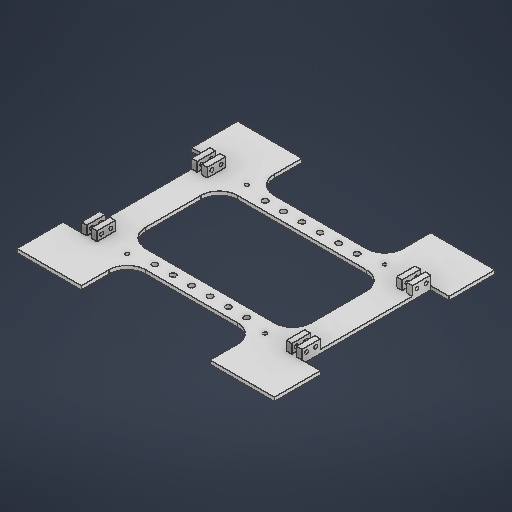
# Autodesk Inventor part: base
Saved by Autodesk Inventor 2026.1 (Build 301233000, 233)
## iProperties
Created: 2025-10-16
Part Number: base
Material: Generic
Document SubType Name: Modeling
Designer: emanuel
Density: 1 g/cm^3
Appearance: Default
Author: emanuel
Autodesk Inventor part; units mm, degrees
ref_plane "YZ Plane" through (0, 0, 0) normal (1, 0, 0) x (0, 1, 0)
ref_plane "XZ Plane" through (0, 0, 0) normal (0, 1, 0) x (-1, 0, 0)
ref_plane "XY Plane" through (0, 0, 0) normal (0, 0, 1) x (1, 0, 0)
sketch "Sketch1" plane through (0, 0, 0) normal (0, 1, 0) x (-1, 0, 0)
  line L0 (0, 0) -> (140, 0)
  line L1 (140, 0) -> (140, -120)
  line L2 (140, -120) -> (0, -120)
  line L3 (0, -120) -> (0, 0)
  line L4 (140, 0) -> (0, 0)
  line L5 (0, 0) -> (0, -25)
  line L6 (0, -25) -> (140, -25)
  line L7 (140, -25) -> (140, 0)
  line L8 (140, -120) -> (0, -120)
  line L9 (0, -120) -> (0, -95)
  line L10 (0, -95) -> (140, -95)
  line L11 (140, -95) -> (140, -120)
  line L12 (140, -25) -> (130, -25)
  line L13 (130, -25) -> (130, -95)
  line L14 (130, -95) -> (140, -95)
  line L15 (140, -95) -> (140, -25)
  line L16 (0, -25) -> (10, -25)
  line L17 (10, -25) -> (10, -95)
  line L18 (10, -95) -> (0, -95)
  line L19 (0, -95) -> (0, -25)
  line L20 (130, -25) -> (115, -25)
  line L21 (115, -25) -> (115, -95)
  line L22 (115, -95) -> (130, -95)
  line L23 (130, -95) -> (130, -25)
  line L24 (10, -95) -> (25, -95)
  line L25 (25, -95) -> (25, -25)
  line L26 (25, -25) -> (10, -25)
  line L27 (10, -25) -> (10, -95)
  line L28 (115, -25) -> (25, -25)
  line L29 (25, -25) -> (25, -35)
  line L30 (25, -35) -> (115, -35)
  line L31 (115, -35) -> (115, -25)
  line L32 (115, -95) -> (25, -95)
  line L33 (25, -95) -> (25, -85)
  line L34 (25, -85) -> (115, -85)
  line L35 (115, -85) -> (115, -95)
  line L36 (115, -30) -> (25, -30)
  line L37 (115, -90) -> (25, -90)
  line L38 (115, -30) -> (105, -30)
  line L39 (105, -30) -> (95, -30)
  line L40 (95, -30) -> (85, -30)
  line L41 (85, -30) -> (75, -30)
  line L42 (75, -30) -> (65, -30)
  line L43 (65, -30) -> (55, -30)
  line L44 (55, -30) -> (45, -30)
  line L45 (45, -30) -> (35, -30)
  line L46 (115, -90) -> (105, -90)
  line L47 (105, -90) -> (95, -90)
  line L48 (95, -90) -> (85, -90)
  line L49 (85, -90) -> (75, -90)
  line L50 (75, -90) -> (65, -90)
  line L51 (65, -90) -> (55, -90)
  line L52 (55, -90) -> (45, -90)
  line L53 (45, -90) -> (35, -90)
  line L54 (35, -90) -> (25, -90)
  circle A0 centre (105, -30) radius 1.5
  circle A1 centre (95, -30) radius 1.5
  circle A2 centre (85, -30) radius 1.5
  circle A3 centre (75, -30) radius 1.5
  circle A4 centre (65, -30) radius 1.5
  circle A5 centre (55, -30) radius 1.5
  circle A6 centre (45, -30) radius 1.5
  circle A7 centre (35, -30) radius 1.5
  circle A8 centre (105, -90) radius 1.5
  circle A9 centre (95, -90) radius 1.5
  circle A10 centre (85, -90) radius 1.5
  circle A11 centre (75, -90) radius 1.5
  circle A12 centre (65, -90) radius 1.5
  circle A13 centre (55, -90) radius 1.5
  circle A14 centre (45, -90) radius 1.5
  circle A15 centre (35, -90) radius 1.5
  line L55 (140, 0) -> (105, 0)
  line L56 (105, 0) -> (105, -25)
  line L57 (105, -25) -> (140, -25)
  line L58 (140, -25) -> (140, 0)
  line L59 (140, -95) -> (105, -95)
  line L60 (105, -95) -> (105, -120)
  line L61 (105, -120) -> (140, -120)
  line L62 (140, -120) -> (140, -95)
  line L63 (0, 0) -> (35, 0)
  line L64 (35, 0) -> (35, -25)
  line L65 (35, -25) -> (0, -25)
  line L66 (0, -25) -> (0, 0)
  line L67 (0, -95) -> (35, -95)
  line L68 (35, -95) -> (35, -120)
  line L69 (35, -120) -> (0, -120)
  line L70 (0, -120) -> (0, -95)
  dimension "d0" = 140
  dimension "d1" = 120
  dimension "d2" = 25
  dimension "d3" = 25
  dimension "d4" = 10
  dimension "d5" = 10
  dimension "d6" = 15
  dimension "d7" = 15
  dimension "d8" = 10
  dimension "d9" = 10
  dimension "d10" = 10
  dimension "d11" = 10
  dimension "d12" = 10
  dimension "d13" = 10
  dimension "d14" = 10
  dimension "d15" = 10
  dimension "d16" = 10
  dimension "d17" = 10
  dimension "d18" = 10
  dimension "d19" = 10
  dimension "d20" = 10
  dimension "d21" = 10
  dimension "d22" = 10
  dimension "d23" = 10
  dimension "d24" = 10
  dimension "d25" = 10
  dimension "d26" = 10
  dimension "d27" = 3
  dimension "d28" = 3
  dimension "d29" = 3
  dimension "d30" = 3
  dimension "d31" = 3
  dimension "d32" = 3
  dimension "d33" = 3
  dimension "d34" = 3
  dimension "d35" = 3
  dimension "d36" = 3
  dimension "d37" = 3
  dimension "d38" = 3
  dimension "d39" = 3
  dimension "d40" = 3
  dimension "d41" = 3
  dimension "d42" = 3
  dimension "d43" = 35
  dimension "d44" = 35
  dimension "d45" = 35
  dimension "d46" = 35
  constraints: 138 end point, 27 equal length, 16 centre point, 16 coincident, 13 horizontal, 13 perpendicular, 12 point on line, 4 midpoint, 22 other
  measures "d0" distance of L1.end L2.end
  measures "d1" distance of L0.end L1.end
  measures "d2" distance of L5.end L4.end
  measures "d3" distance of L8.end L9.end
  measures "d4" distance of L14.end L13.end
  measures "d5" distance of L17.end L18.end
  measures "d6" distance of L22.end L21.end
  measures "d7" distance of L26.end L25.end
  measures "d8" distance of L29.end L28.end
  measures "d9" distance of L32.end L33.end
  measures "d10" distance of L38.start L38.end
  measures "d11" distance of L38.end L39.end
  measures "d12" distance of L39.end L40.end
  measures "d13" distance of L40.end L41.end
  measures "d14" distance of L41.end L42.end
  measures "d15" distance of L42.end L43.end
  measures "d16" distance of L43.end L44.end
  measures "d17" distance of L44.end L45.end
  measures "d18" distance of L46.start L46.end
  measures "d19" distance of L46.end L47.end
  measures "d20" distance of L47.end L48.end
  measures "d21" distance of L48.end L49.end
  measures "d22" distance of L49.end L50.end
  measures "d23" distance of L50.end L51.end
  measures "d24" distance of L51.end L52.end
  measures "d25" distance of L52.end L53.end
  measures "d26" distance of L53.end L54.end
  measures "d27" diameter of A0
  measures "d28" diameter of A1
  measures "d29" diameter of A2
  measures "d30" diameter of A3
  measures "d31" diameter of A4
  measures "d32" diameter of A5
  measures "d33" diameter of A6
  measures "d34" diameter of A7
  measures "d35" diameter of A8
  measures "d36" diameter of A9
  measures "d37" diameter of A10
  measures "d38" diameter of A11
  measures "d39" diameter of A12
  measures "d40" diameter of A13
  measures "d41" diameter of A14
  measures "d42" diameter of A15
  measures "d43" distance of L57.end L56.end
  measures "d44" distance of L61.end L60.end
  measures "d45" distance of L64.end L65.end
  measures "d46" distance of L68.end L69.end
extrude "Extrusion1" add sketch "Sketch1" along normal blind 2 contours L0 L64 L6 L3 | L0 L1 L6 L56 | L6 L21 L36 A0 A1 A2 A3 A4 A5 A6 A7 L25 | L10 L68 L2 L3 | L6 L25 L10 L17 | L6 L13 L10 L21 | L36 A7 A6 A5 A4 A3 A2 A1 A0 L21 L30 L25 | L25 L37 A15 A14 A13 A12 A11 A10 A9 A8 L21 L10 | L1 L2 L60 L10 | A7 L36 | L36 A7 | L25 L34 L21 L37 A8 A9 A10 A11 A12 A13 A14 A15 | A0 L36 | L36 A0 | A15 L37 | L37 A15 | A8 L37 | L37 A8
fillet "Fillet1" radius 10 8 edges at (-105, 1, -25) (-115, 1, -85) (-25, 1, -85) (-25, 1, -35) (-115, 1, -35) (-35, 1, -95) (-105, 1, -95) (-35, 1, -25)
sketch "Sketch2" plane through (0, 2, 0) normal (0, 1, 0) x (1, 0, 0)
  line L0 (-130, 95) -> (-130, 25) projected
  line L1 (-130, 25) -> (-127, 25)
  line L2 (-127, 25) -> (-127, 95)
  line L3 (-127, 95) -> (-130, 95)
  line L4 (-130, 95) -> (-130, 25)
  line L5 (-127, 25) -> (-124.5, 25)
  line L6 (-124.5, 25) -> (-124.5, 95)
  line L7 (-124.5, 95) -> (-127, 95)
  line L8 (-127, 95) -> (-127, 25)
  line L9 (-124.5, 25) -> (-121.5, 25)
  line L10 (-121.5, 25) -> (-121.5, 95)
  line L11 (-121.5, 95) -> (-124.5, 95)
  line L12 (-124.5, 95) -> (-124.5, 25)
  line L13 (-10, 25) -> (-10, 95) projected
  line L14 (-10, 25) -> (-13, 25)
  line L15 (-13, 25) -> (-13, 95)
  line L16 (-13, 95) -> (-10, 95)
  line L17 (-10, 95) -> (-10, 25)
  line L18 (-13, 25) -> (-15.5, 25)
  line L19 (-15.5, 25) -> (-15.5, 95)
  line L20 (-15.5, 95) -> (-13, 95)
  line L21 (-13, 95) -> (-13, 25)
  line L22 (-15.5, 25) -> (-18.5, 25)
  line L23 (-18.5, 25) -> (-18.5, 95)
  line L24 (-18.5, 95) -> (-15.5, 95)
  line L25 (-15.5, 95) -> (-15.5, 25)
  line L26 (-130, 25) -> (-121.5, 25)
  line L27 (-121.5, 25) -> (-121.5, 35)
  line L28 (-121.5, 35) -> (-130, 35)
  line L29 (-130, 35) -> (-130, 25)
  line L30 (-130, 95) -> (-121.5, 95)
  line L31 (-121.5, 95) -> (-121.5, 85)
  line L32 (-121.5, 85) -> (-130, 85)
  line L33 (-130, 85) -> (-130, 95)
  line L34 (-18.5, 25) -> (-10, 25)
  line L35 (-10, 25) -> (-10, 35)
  line L36 (-10, 35) -> (-18.5, 35)
  line L37 (-18.5, 35) -> (-18.5, 25)
  line L38 (-18.5, 95) -> (-10, 95)
  line L39 (-10, 95) -> (-10, 85)
  line L40 (-10, 85) -> (-18.5, 85)
  line L41 (-18.5, 85) -> (-18.5, 95)
  line L42 (-130, 25) -> (-127, 25)
  line L43 (-127, 25) -> (-127, 35)
  line L44 (-127, 35) -> (-130, 35)
  line L45 (-130, 35) -> (-130, 25)
  line L46 (-18.5, 25) -> (-15.5, 25)
  line L47 (-15.5, 25) -> (-15.5, 35)
  line L48 (-15.5, 35) -> (-18.5, 35)
  line L49 (-18.5, 35) -> (-18.5, 25)
  point P0 (0, 0)
  point P1 (-124.5, 35)
  point P2 (-124.5, 85)
  point P3 (-127, 85)
  point P4 (-13, 35)
  point P5 (-13, 85)
  point P6 (-15.5, 85)
  dimension "d50" = 3
  dimension "d51" = 2.5
  dimension "d52" = 3
  dimension "d53" = 3
  dimension "d54" = 2.5
  dimension "d55" = 3
  dimension "d56" = 10
  dimension "d57" = 10
  dimension "d58" = 10
  dimension "d59" = 10
  constraints: 96 end point, 24 parallel, 13 point on line, 12 horizontal, 12 perpendicular
  measures "d50" distance of L3.end L2.end
  measures "d51" distance of L7.end L6.end
  measures "d52" distance of L11.end L10.end
  measures "d53" distance of L15.end L16.end
  measures "d54" distance of L19.end L20.end
  measures "d55" distance of L23.end L24.end
  measures "d56" distance of L27.end L26.end
  measures "d57" distance of L30.end L31.end
  measures "d58" distance of L35.end L34.end
  measures "d59" distance of L38.end L39.end
extrude "Extrusion2" add sketch "Sketch2" along normal blind 5 contours L3 L2 L32 L0 | L28 L2 L1 L0 | L11 L10 L32 L6 | L28 L10 L9 L6 | L14 L15 L36 L13 | L40 L15 L16 L13 | L22 L23 L36 L19 | L40 L23 L24 L19
sketch "Sketch3" plane through (-10, 0, -25) normal (1, 0, 0) x (0, 0, -1)
  line L0 (0, 7) -> (10, 7) projected
  line L1 (0, 7) -> (2.5, 7)
  line L2 (2.5, 7) -> (2.5, 4.5)
  line L3 (2.5, 4.5) -> (0, 4.5)
  line L4 (0, 4.5) -> (0, 7)
  line L5 (2.5, 4.5) -> (7.5, 4.5)
  circle A0 centre (2.5, 4.5) radius 1
  circle A1 centre (7.5, 4.5) radius 1
  line L6 (60, 7) -> (70, 7) projected
  line L7 (60, 7) -> (62.5, 7)
  line L8 (62.5, 7) -> (62.5, 4.5)
  line L9 (62.5, 4.5) -> (60, 4.5)
  line L10 (60, 4.5) -> (60, 7)
  line L11 (62.5, 4.5) -> (67.5, 4.5)
  circle A2 centre (67.5, 4.5) radius 1
  circle A3 centre (62.5, 4.5) radius 1
  point P0 (-25, 0)
  dimension "d62" = 2.5
  dimension "d63" = 2.5
  dimension "d64" = 5
  dimension "d65" = 2
  dimension "d66" = 2
  dimension "d67" = 2.5
  dimension "d68" = 2.5
  dimension "d69" = 5
  dimension "d70" = 2
  dimension "d71" = 2
  constraints: 20 end point, 4 centre point, 4 coincident, 4 horizontal, 4 parallel, 2 perpendicular
  measures "d62" distance of L2.end L3.end
  measures "d63" distance of L1.end L2.end
  measures "d64" distance of L2.end L5.end
  measures "d65" diameter of A0
  measures "d66" diameter of A1
  measures "d67" distance of L8.end L9.end
  measures "d68" distance of L7.end L8.end
  measures "d69" distance of L8.end L11.end
  measures "d70" diameter of A2
  measures "d71" diameter of A3
extrude "Extrusion3" cut sketch "Sketch3" against normal up to surface (120 mm away) contours A0 L5 L2 | L2 L3 A0 | L3 L5 A0 | A1 | A3 L11 L8 | L8 L9 A3 | L9 L11 A3 | A2
sketch "Sketch4" plane through (0, 2, 0) normal (0, 1, 0) x (1, 0, 0)
  line L0 (0, 95) -> (0, 120) projected
  line L1 (0, 120) -> (-32.5, 120)
  line L2 (-32.5, 120) -> (-32.5, 92.5)
  line L3 (-32.5, 92.5) -> (0, 92.5)
  line L4 (0, 92.5) -> (0, 120)
  line L5 (-35, 0) -> (0, 0) projected
  line L6 (0, 0) -> (-32.5, 0)
  line L7 (-32.5, 0) -> (-32.5, 27.5)
  line L8 (-32.5, 27.5) -> (0, 27.5)
  line L9 (0, 27.5) -> (0, 0)
  line L10 (-140, 120) -> (-140, 95) projected
  line L11 (-140, 120) -> (-107.5, 120)
  line L12 (-107.5, 120) -> (-107.5, 92.5)
  line L13 (-107.5, 92.5) -> (-140, 92.5)
  line L14 (-140, 92.5) -> (-140, 120)
  line L15 (-140, 0) -> (-107.5, 0)
  line L16 (-107.5, 0) -> (-107.5, 27.5)
  line L17 (-107.5, 27.5) -> (-140, 27.5)
  line L18 (-140, 27.5) -> (-140, 0)
  circle A0 centre (-107.5, 27.5) radius 1
  circle A1 centre (-32.5, 27.5) radius 1
  circle A2 centre (-32.5, 92.5) radius 1
  circle A3 centre (-107.5, 92.5) radius 1
  dimension "d74" = 32.5
  dimension "d75" = 27.5
  dimension "d76" = 32.5
  dimension "d77" = 27.5
  dimension "d78" = 32.5
  dimension "d79" = 27.5
  dimension "d80" = 32.5
  dimension "d81" = 27.5
  dimension "d82" = 2
  dimension "d83" = 2
  dimension "d84" = 2
  dimension "d85" = 2
  constraints: 32 end point, 8 parallel, 4 centre point, 4 coincident, 4 horizontal, 4 perpendicular, 2 point on line
  measures "d74" distance of L3.end L2.end
  measures "d75" distance of L2.end L1.end
  measures "d76" distance of L7.end L8.end
  measures "d77" distance of L6.end L7.end
  measures "d78" distance of L12.end L13.end
  measures "d79" distance of L11.end L12.end
  measures "d80" distance of L17.end L16.end
  measures "d81" distance of L16.end L15.end
  measures "d82" diameter of A0
  measures "d83" diameter of A1
  measures "d84" diameter of A2
  measures "d85" diameter of A3
extrude "Extrusion4" cut sketch "Sketch4" against normal blind 10 contours A2 L2 L3 | L3 L2 A2 | A1 L8 L7 | L7 L8 A1 | A3 L13 L12 | L12 L13 A3 | A0 L17 L16 | L16 L17 A0
body "Solid1"
